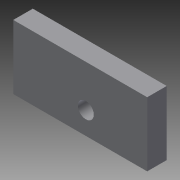
# Autodesk Inventor part: FrameEndSpacer_NERDS
Saved by Autodesk Inventor 2014 (Build 180170000, 170)
## iProperties
Created: 2016-01-30
Part Number: FrameEndSpacer_NERDS
Material: Generic
Document SubType Name: Modeling
Designer: bermudezr
Density: 1 g/cm^3
Appearance: Default
Author: bermudezr
Autodesk Inventor part; units mm, degrees
ref_plane "YZ Plane" through (0, 0, 0) normal (1, 0, 0) x (0, 1, 0)
ref_plane "XZ Plane" through (0, 0, 0) normal (0, 1, 0) x (-1, 0, 0)
ref_plane "XY Plane" through (0, 0, 0) normal (0, 0, 1) x (1, 0, 0)
sketch "Sketch1" plane through (0, 0, 0) normal (0, 0, 1) x (1, 0, 0)
  line L0 (-58.6409, 36.9404) -> (93.7591, 36.9404)
  line L1 (93.7591, 36.9404) -> (93.7591, -36.0846)
  line L2 (93.7591, -36.0846) -> (-58.6409, -36.0846)
  line L3 (-58.6409, -36.0846) -> (-58.6409, 36.9404)
  point P0 (0, 0)
  dimension "d0" = 152.4
  dimension "d1" = 73.025
  constraints: 8 end point, 2 parallel, 1 horizontal, 1 perpendicular
  measures "d0" distance of L0.start L0.end
  measures "d1" distance of L2.end L0.start
extrude "Extrusion1" add sketch "Sketch1" along normal blind 22.225
sketch "Sketch2" plane through (0, 0, 22.225) normal (0, 0, 1) x (1, 0, 0)
  line L0 (-58.6409, 36.9404) -> (-58.6409, -36.0846) projected
  line L1 (-58.6409, -36.0846) -> (93.7591, -36.0846) projected
  circle A0 centre (23.9091, -10.6846) radius 9.092
  point P0 (0, 0)
  dimension "d4" = 82.55
  dimension "d5" = 25.4
  constraints: 1 centre point
  measures "d4" distance from line of A0.centre L0
  measures "d5" distance from line of L1 A0.centre
extrude "Extrusion2" cut sketch "Sketch2" against normal blind 22.225
body "Solid1"
